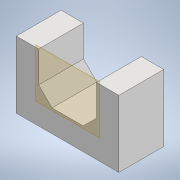
# Autodesk Inventor part: UpperJawsuuport
Saved by Autodesk Inventor 2022 (Build 260153000, 153)
## iProperties
Created: 2021-11-02
Part Number: UpperJawsuuport
Material: Genérico
Document SubType Name: Modeling
Designer: JK
Density: 1 g/cm^3
Appearance: Valor por defecto
Author: JK
Autodesk Inventor part; units mm, degrees
ref_plane "YZ Plane" through (0, 0, 0) normal (1, 0, 0) x (0, 1, 0)
ref_plane "XZ Plane" through (0, 0, 0) normal (0, 1, 0) x (-1, 0, 0)
ref_plane "Plano de trabajo1" through (0, -0.4184, 0) normal (0, 0, 1) x (1, 0, 0)
sketch "Boceto1" plane through (0, -0.4184, 0) normal (0, 0, 1) x (1, 0, 0)
  line L0 (51.8, 12.5012) -> (51.8, 40.2184) projected
  line L1 (51.8, 40.2184) -> (0.2, 40.2184) projected
  line L2 (0.2, 40.2184) -> (0.2, 12.5012) projected
  line L3 (0.2, 12.5012) -> (12.0828, 0.6184) projected
  line L4 (12.0828, 0.6184) -> (39.9172, 0.6184) projected
  line L5 (39.9172, 0.6184) -> (51.8, 12.5012) projected
  circle A0 centre (26, 20.4184) radius 14.2 projected
  line L6 (71.8, 40.2184) -> (-19.8, 40.2184)
  line L7 (-19.8, 40.2184) -> (-19.8, -19.3816)
  line L8 (-19.8, -19.3816) -> (71.8, -19.3816)
  line L9 (71.8, -19.3816) -> (71.8, 40.2184)
  point P0 (0, 0.4184)
  point P1 (0.2, 40.2184)
  point P2 (51.8, 40.2184)
  dimension "d0" = 20
  dimension "d1" = 20
  dimension "d2" = 20
  constraints: 8 end point, 2 parallel, 1 horizontal, 1 perpendicular, 1 point on line
  measures "d0" distance between parallel lines of L0 L9
  measures "d1" distance between parallel lines of L7 L2
  measures "d2" distance between parallel lines of L8 L4
extrude "Extrusión1" add sketch "Boceto1" against normal blind 40 contours L0 L6 L9 L8 L7 L2 L3 L4 L5
sketch "Boceto2" plane through (0, -0.4184, 0) normal (0, 0, 1) x (1, 0, 0)
  line L0 (39.9172, 0.6184) -> (12.0828, 0.6184) projected
  line L1 (12.0828, 0.6184) -> (0.2, 12.5012) projected
  line L2 (0.2, 12.5012) -> (0.2, 40.2184) projected
  line L3 (0.2, 40.2184) -> (-19.8, 40.2184) projected
  line L4 (-19.8, 40.2184) -> (-19.8, -19.3816) projected
  line L5 (-19.8, -19.3816) -> (71.8, -19.3816) projected
  line L6 (71.8, -19.3816) -> (71.8, 40.2184) projected
  line L7 (71.8, 40.2184) -> (51.8, 40.2184) projected
  line L8 (51.8, 40.2184) -> (51.8, 12.5012) projected
  line L9 (51.8, 12.5012) -> (39.9172, 0.6184) projected
  point P0 (0, 0.4184)
extrude "Extrusión2" add sketch "Boceto2" along normal blind 10 and the other way blind 50
sketch "Boceto3" plane through (-19.8, 39.8, -50) normal (0, 1, 0) x (1, 0, 0)
  circle A0 centre (5.8, -10) radius 2.7
  circle A1 centre (5.8, -50) radius 2.7
  circle A2 centre (85.8, -10) radius 2.7
  circle A3 centre (85.8, -50) radius 2.7
  line L0 (0, 0) -> (20, 0) projected
  line L1 (59.7172, -60) -> (31.8828, -60) projected
  line L2 (45.8, -60) -> (45.8, 0)
  point P0 (19.8, -50)
  dimension "d9" = 80
  dimension "d10" = 5.4
  dimension "d11" = 40
  dimension "d12" = 10
  dimension "d13" = 40
  constraints: 4 centre point, 3 equal radius, 2 end point, 2 horizontal alignment, 2 vertical alignment, 1 midpoint, 1 vertical
  measures "d9" distance of A2.centre A0.centre
  measures "d10" diameter of A0
  measures "d11" distance of A0.centre A1.centre
  measures "d12" distance from line of L0 A0.centre
  measures "d13" distance from line of L2 A0.centre
extrude "Extrusión3" cut sketch "Boceto3" against normal through all
